Autodesk Fusion 360 part; units mm, degrees
(part 3 of 7)
sketch "Sketch8" plane through (0, 0, 0) normal (0, 0, 1) x (1, 0, 0)
  arc A0 (-0.8091, 5.4143) -> (-0.6399, 5.6347) centre (-0.8386, 5.6121) ccw
  arc A1 (0.6399, 5.6347) -> (0.8091, 5.4143) centre (0.8386, 5.6121) ccw
  line L0 (0.6399, 5.6347) -> (0.6786, 5.9756)
  spline S0 degree 5 poles (0.6786, 5.9756) (0.679, 5.9791) (0.6797, 5.9859) (0.6804, 5.9963) (0.6808, 6.0101) (0.6806, 6.0275) (0.6798, 6.0448) (0.6786, 6.0622) (0.6773, 6.0796) (0.6758, 6.0971) (0.6742, 6.1145) (0.6724, 6.132) (0.6704, 6.1495) (0.6682, 6.167) (0.6656, 6.1845) (0.6628, 6.202) (0.6598, 6.2196) (0.6566, 6.2371) (0.6532, 6.2546) (0.6497, 6.2722) (0.646, 6.2897) (0.6422, 6.3073) (0.6382, 6.3249) (0.634, 6.3424) (0.6297, 6.36) (0.6252, 6.3776) (0.6205, 6.3951) (0.6157, 6.4127) (0.6108, 6.4303) (0.6057, 6.4478) (0.6004, 6.4654) (0.595, 6.4829) (0.5895, 6.5005) (0.5838, 6.5181) (0.578, 6.5356) (0.5721, 6.5532) (0.566, 6.5707) (0.5598, 6.5882) (0.5535, 6.6058) (0.547, 6.6233) (0.5404, 6.6408) (0.5336, 6.6583) (0.5268, 6.6758) (0.5198, 6.6933) (0.5127, 6.7108) (0.5055, 6.7283) (0.4981, 6.7457) (0.4906, 6.7632) (0.483, 6.7806) (0.4753, 6.7981) (0.4675, 6.8155) (0.4595, 6.8329) (0.4514, 6.8503) (0.4432, 6.8677) (0.4349, 6.8851) (0.4265, 6.9024) (0.418, 6.9198) (0.4093, 6.9371) (0.4006, 6.9544) (0.3917, 6.9717) (0.3827, 6.989) (0.3736, 7.0063) (0.3644, 7.0235) (0.355, 7.0408) (0.3456, 7.058) (0.3361, 7.0752) (0.3264, 7.0924) (0.3167, 7.1095) (0.3068, 7.1267) (0.2968, 7.1438) (0.2867, 7.1609) (0.2786, 7.1746) (0.2724, 7.1848) (0.2683, 7.1917) (0.2662, 7.1951) knots 0 0 0 0 0 0 0.01428571 0.02857143 0.04285714 0.05714286 0.07142857 0.08571429 0.1 0.11428571 0.12857143 0.14285714 0.15714286 0.17142857 0.18571429 0.2 0.21428571 0.22857143 0.24285714 0.25714286 0.27142857 0.28571429 0.3 0.31428571 0.32857143 0.34285714 0.35714286 0.37142857 0.38571429 0.4 0.41428571 0.42857143 0.44285714 0.45714286 0.47142857 0.48571429 0.5 0.51428571 0.52857143 0.54285714 0.55714286 0.57142857 0.58571429 0.6 0.61428571 0.62857143 0.64285714 0.65714286 0.67142857 0.68571429 0.7 0.71428571 0.72857143 0.74285714 0.75714286 0.77142857 0.78571429 0.8 0.81428571 0.82857143 0.84285714 0.85714286 0.87142857 0.88571429 0.9 0.91428571 0.92857143 0.94285714 0.95714286 0.97142857 0.98571429 1 1 1 1 1 1
  line L1 (-0.6786, 5.9756) -> (-0.6399, 5.6347)
  spline S1 degree 5 poles (-0.6786, 5.9756) (-0.679, 5.9791) (-0.6797, 5.9859) (-0.6804, 5.9963) (-0.6808, 6.0101) (-0.6806, 6.0275) (-0.6798, 6.0448) (-0.6786, 6.0622) (-0.6773, 6.0796) (-0.6758, 6.0971) (-0.6742, 6.1145) (-0.6724, 6.132) (-0.6704, 6.1495) (-0.6682, 6.167) (-0.6656, 6.1845) (-0.6628, 6.202) (-0.6598, 6.2196) (-0.6566, 6.2371) (-0.6532, 6.2546) (-0.6497, 6.2722) (-0.646, 6.2897) (-0.6422, 6.3073) (-0.6382, 6.3249) (-0.634, 6.3424) (-0.6297, 6.36) (-0.6252, 6.3776) (-0.6205, 6.3951) (-0.6157, 6.4127) (-0.6108, 6.4303) (-0.6057, 6.4478) (-0.6004, 6.4654) (-0.595, 6.4829) (-0.5895, 6.5005) (-0.5838, 6.5181) (-0.578, 6.5356) (-0.5721, 6.5532) (-0.566, 6.5707) (-0.5598, 6.5882) (-0.5535, 6.6058) (-0.547, 6.6233) (-0.5404, 6.6408) (-0.5336, 6.6583) (-0.5268, 6.6758) (-0.5198, 6.6933) (-0.5127, 6.7108) (-0.5055, 6.7283) (-0.4981, 6.7457) (-0.4906, 6.7632) (-0.483, 6.7806) (-0.4753, 6.7981) (-0.4675, 6.8155) (-0.4595, 6.8329) (-0.4514, 6.8503) (-0.4432, 6.8677) (-0.4349, 6.8851) (-0.4265, 6.9024) (-0.418, 6.9198) (-0.4093, 6.9371) (-0.4006, 6.9544) (-0.3917, 6.9717) (-0.3827, 6.989) (-0.3736, 7.0063) (-0.3644, 7.0235) (-0.355, 7.0408) (-0.3456, 7.058) (-0.3361, 7.0752) (-0.3264, 7.0924) (-0.3167, 7.1095) (-0.3068, 7.1267) (-0.2968, 7.1438) (-0.2867, 7.1609) (-0.2786, 7.1746) (-0.2724, 7.1848) (-0.2683, 7.1917) (-0.2662, 7.1951) knots 0 0 0 0 0 0 0.01428571 0.02857143 0.04285714 0.05714286 0.07142857 0.08571429 0.1 0.11428571 0.12857143 0.14285714 0.15714286 0.17142857 0.18571429 0.2 0.21428571 0.22857143 0.24285714 0.25714286 0.27142857 0.28571429 0.3 0.31428571 0.32857143 0.34285714 0.35714286 0.37142857 0.38571429 0.4 0.41428571 0.42857143 0.44285714 0.45714286 0.47142857 0.48571429 0.5 0.51428571 0.52857143 0.54285714 0.55714286 0.57142857 0.58571429 0.6 0.61428571 0.62857143 0.64285714 0.65714286 0.67142857 0.68571429 0.7 0.71428571 0.72857143 0.74285714 0.75714286 0.77142857 0.78571429 0.8 0.81428571 0.82857143 0.84285714 0.85714286 0.87142857 0.88571429 0.9 0.91428571 0.92857143 0.94285714 0.95714286 0.97142857 0.98571429 1 1 1 1 1 1
  spline S2 degree 5 poles (-0.2662, 7.1951) (-0.2683, 7.1917) (-0.2724, 7.1848) (-0.2786, 7.1746) (-0.2867, 7.1609) (-0.2968, 7.1438) (-0.3068, 7.1267) (-0.3167, 7.1095) (-0.3264, 7.0924) (-0.3361, 7.0752) (-0.3456, 7.058) (-0.355, 7.0408) (-0.3644, 7.0235) (-0.3736, 7.0063) (-0.3827, 6.989) (-0.3917, 6.9717) (-0.4006, 6.9544) (-0.4093, 6.9371) (-0.418, 6.9198) (-0.4265, 6.9024) (-0.4349, 6.8851) (-0.4432, 6.8677) (-0.4514, 6.8503) (-0.4595, 6.8329) (-0.4675, 6.8155) (-0.4753, 6.7981) (-0.483, 6.7806) (-0.4906, 6.7632) (-0.4981, 6.7457) (-0.5055, 6.7283) (-0.5127, 6.7108) (-0.5198, 6.6933) (-0.5268, 6.6758) (-0.5336, 6.6583) (-0.5404, 6.6408) (-0.547, 6.6233) (-0.5535, 6.6058) (-0.5598, 6.5882) (-0.566, 6.5707) (-0.5721, 6.5532) (-0.578, 6.5356) (-0.5838, 6.5181) (-0.5895, 6.5005) (-0.595, 6.4829) (-0.6004, 6.4654) (-0.6057, 6.4478) (-0.6108, 6.4303) (-0.6157, 6.4127) (-0.6205, 6.3951) (-0.6252, 6.3776) (-0.6297, 6.36) (-0.634, 6.3424) (-0.6382, 6.3249) (-0.6422, 6.3073) (-0.646, 6.2897) (-0.6497, 6.2722) (-0.6532, 6.2546) (-0.6566, 6.2371) (-0.6598, 6.2196) (-0.6628, 6.202) (-0.6656, 6.1845) (-0.6682, 6.167) (-0.6704, 6.1495) (-0.6724, 6.132) (-0.6742, 6.1145) (-0.6758, 6.0971) (-0.6773, 6.0796) (-0.6786, 6.0622) (-0.6798, 6.0448) (-0.6806, 6.0275) (-0.6808, 6.0101) (-0.6804, 5.9963) (-0.6797, 5.9859) (-0.679, 5.9791) (-0.6786, 5.9756) knots -1 -1 -1 -1 -1 -1 -0.98571429 -0.97142857 -0.95714286 -0.94285714 -0.92857143 -0.91428571 -0.9 -0.88571429 -0.87142857 -0.85714286 -0.84285714 -0.82857143 -0.81428571 -0.8 -0.78571429 -0.77142857 -0.75714286 -0.74285714 -0.72857143 -0.71428571 -0.7 -0.68571429 -0.67142857 -0.65714286 -0.64285714 -0.62857143 -0.61428571 -0.6 -0.58571429 -0.57142857 -0.55714286 -0.54285714 -0.52857143 -0.51428571 -0.5 -0.48571429 -0.47142857 -0.45714286 -0.44285714 -0.42857143 -0.41428571 -0.4 -0.38571429 -0.37142857 -0.35714286 -0.34285714 -0.32857143 -0.31428571 -0.3 -0.28571429 -0.27142857 -0.25714286 -0.24285714 -0.22857143 -0.21428571 -0.2 -0.18571429 -0.17142857 -0.15714286 -0.14285714 -0.12857143 -0.11428571 -0.1 -0.08571429 -0.07142857 -0.05714286 -0.04285714 -0.02857143 -0.01428571 0 0 0 0 0 0
  spline S3 degree 5 poles (-0.2662, 7.1951) (-0.2683, 7.1917) (-0.2724, 7.1848) (-0.2786, 7.1746) (-0.2867, 7.1609) (-0.2968, 7.1438) (-0.3068, 7.1267) (-0.3167, 7.1095) (-0.3264, 7.0924) (-0.3361, 7.0752) (-0.3456, 7.058) (-0.355, 7.0408) (-0.3644, 7.0235) (-0.3736, 7.0063) (-0.3827, 6.989) (-0.3917, 6.9717) (-0.4006, 6.9544) (-0.4093, 6.9371) (-0.418, 6.9198) (-0.4265, 6.9024) (-0.4349, 6.8851) (-0.4432, 6.8677) (-0.4514, 6.8503) (-0.4595, 6.8329) (-0.4675, 6.8155) (-0.4753, 6.7981) (-0.483, 6.7806) (-0.4906, 6.7632) (-0.4981, 6.7457) (-0.5055, 6.7283) (-0.5127, 6.7108) (-0.5198, 6.6933) (-0.5268, 6.6758) (-0.5336, 6.6583) (-0.5404, 6.6408) (-0.547, 6.6233) (-0.5535, 6.6058) (-0.5598, 6.5882) (-0.566, 6.5707) (-0.5721, 6.5532) (-0.578, 6.5356) (-0.5838, 6.5181) (-0.5895, 6.5005) (-0.595, 6.4829) (-0.6004, 6.4654) (-0.6057, 6.4478) (-0.6108, 6.4303) (-0.6157, 6.4127) (-0.6205, 6.3951) (-0.6252, 6.3776) (-0.6297, 6.36) (-0.634, 6.3424) (-0.6382, 6.3249) (-0.6422, 6.3073) (-0.646, 6.2897) (-0.6497, 6.2722) (-0.6532, 6.2546) (-0.6566, 6.2371) (-0.6598, 6.2196) (-0.6628, 6.202) (-0.6656, 6.1845) (-0.6682, 6.167) (-0.6704, 6.1495) (-0.6724, 6.132) (-0.6742, 6.1145) (-0.6758, 6.0971) (-0.6773, 6.0796) (-0.6786, 6.0622) (-0.6798, 6.0448) (-0.6806, 6.0275) (-0.6808, 6.0101) (-0.6804, 5.9963) (-0.6797, 5.9859) (-0.679, 5.9791) (-0.6786, 5.9756) knots -1 -1 -1 -1 -1 -1 -0.98571429 -0.97142857 -0.95714286 -0.94285714 -0.92857143 -0.91428571 -0.9 -0.88571429 -0.87142857 -0.85714286 -0.84285714 -0.82857143 -0.81428571 -0.8 -0.78571429 -0.77142857 -0.75714286 -0.74285714 -0.72857143 -0.71428571 -0.7 -0.68571429 -0.67142857 -0.65714286 -0.64285714 -0.62857143 -0.61428571 -0.6 -0.58571429 -0.57142857 -0.55714286 -0.54285714 -0.52857143 -0.51428571 -0.5 -0.48571429 -0.47142857 -0.45714286 -0.44285714 -0.42857143 -0.41428571 -0.4 -0.38571429 -0.37142857 -0.35714286 -0.34285714 -0.32857143 -0.31428571 -0.3 -0.28571429 -0.27142857 -0.25714286 -0.24285714 -0.22857143 -0.21428571 -0.2 -0.18571429 -0.17142857 -0.15714286 -0.14285714 -0.12857143 -0.11428571 -0.1 -0.08571429 -0.07142857 -0.05714286 -0.04285714 -0.02857143 -0.01428571 0 0 0 0 0 0
  arc A2 (0.2662, 7.1951) -> (-0.2662, 7.1951) centre (0, 0) ccw
  arc A3 (-0.8091, 5.4143) -> (-0.6399, 5.6347) centre (-0.8386, 5.6121) ccw
  line L2 (-0.6399, 5.6347) -> (-0.6786, 5.9756)
  spline S4 degree 5 poles (-0.6786, 5.9756) (-0.679, 5.9791) (-0.6797, 5.9859) (-0.6804, 5.9963) (-0.6808, 6.0101) (-0.6806, 6.0275) (-0.6798, 6.0448) (-0.6786, 6.0622) (-0.6773, 6.0796) (-0.6758, 6.0971) (-0.6742, 6.1145) (-0.6724, 6.132) (-0.6704, 6.1495) (-0.6682, 6.167) (-0.6656, 6.1845) (-0.6628, 6.202) (-0.6598, 6.2196) (-0.6566, 6.2371) (-0.6532, 6.2546) (-0.6497, 6.2722) (-0.646, 6.2897) (-0.6422, 6.3073) (-0.6382, 6.3249) (-0.634, 6.3424) (-0.6297, 6.36) (-0.6252, 6.3776) (-0.6205, 6.3951) (-0.6157, 6.4127) (-0.6108, 6.4303) (-0.6057, 6.4478) (-0.6004, 6.4654) (-0.595, 6.4829) (-0.5895, 6.5005) (-0.5838, 6.5181) (-0.578, 6.5356) (-0.5721, 6.5532) (-0.566, 6.5707) (-0.5598, 6.5882) (-0.5535, 6.6058) (-0.547, 6.6233) (-0.5404, 6.6408) (-0.5336, 6.6583) (-0.5268, 6.6758) (-0.5198, 6.6933) (-0.5127, 6.7108) (-0.5055, 6.7283) (-0.4981, 6.7457) (-0.4906, 6.7632) (-0.483, 6.7806) (-0.4753, 6.7981) (-0.4675, 6.8155) (-0.4595, 6.8329) (-0.4514, 6.8503) (-0.4432, 6.8677) (-0.4349, 6.8851) (-0.4265, 6.9024) (-0.418, 6.9198) (-0.4093, 6.9371) (-0.4006, 6.9544) (-0.3917, 6.9717) (-0.3827, 6.989) (-0.3736, 7.0063) (-0.3644, 7.0235) (-0.355, 7.0408) (-0.3456, 7.058) (-0.3361, 7.0752) (-0.3264, 7.0924) (-0.3167, 7.1095) (-0.3068, 7.1267) (-0.2968, 7.1438) (-0.2867, 7.1609) (-0.2786, 7.1746) (-0.2724, 7.1848) (-0.2683, 7.1917) (-0.2662, 7.1951) knots 0 0 0 0 0 0 0.01428571 0.02857143 0.04285714 0.05714286 0.07142857 0.08571429 0.1 0.11428571 0.12857143 0.14285714 0.15714286 0.17142857 0.18571429 0.2 0.21428571 0.22857143 0.24285714 0.25714286 0.27142857 0.28571429 0.3 0.31428571 0.32857143 0.34285714 0.35714286 0.37142857 0.38571429 0.4 0.41428571 0.42857143 0.44285714 0.45714286 0.47142857 0.48571429 0.5 0.51428571 0.52857143 0.54285714 0.55714286 0.57142857 0.58571429 0.6 0.61428571 0.62857143 0.64285714 0.65714286 0.67142857 0.68571429 0.7 0.71428571 0.72857143 0.74285714 0.75714286 0.77142857 0.78571429 0.8 0.81428571 0.82857143 0.84285714 0.85714286 0.87142857 0.88571429 0.9 0.91428571 0.92857143 0.94285714 0.95714286 0.97142857 0.98571429 1 1 1 1 1 1
  arc A4 (0.2662, 7.1951) -> (-0.2662, 7.1951) centre (0, 0) ccw
  spline S5 degree 5 poles (0.6786, 5.9756) (0.679, 5.9791) (0.6797, 5.9859) (0.6804, 5.9963) (0.6808, 6.0101) (0.6806, 6.0275) (0.6798, 6.0448) (0.6786, 6.0622) (0.6773, 6.0796) (0.6758, 6.0971) (0.6742, 6.1145) (0.6724, 6.132) (0.6704, 6.1495) (0.6682, 6.167) (0.6656, 6.1845) (0.6628, 6.202) (0.6598, 6.2196) (0.6566, 6.2371) (0.6532, 6.2546) (0.6497, 6.2722) (0.646, 6.2897) (0.6422, 6.3073) (0.6382, 6.3249) (0.634, 6.3424) (0.6297, 6.36) (0.6252, 6.3776) (0.6205, 6.3951) (0.6157, 6.4127) (0.6108, 6.4303) (0.6057, 6.4478) (0.6004, 6.4654) (0.595, 6.4829) (0.5895, 6.5005) (0.5838, 6.5181) (0.578, 6.5356) (0.5721, 6.5532) (0.566, 6.5707) (0.5598, 6.5882) (0.5535, 6.6058) (0.547, 6.6233) (0.5404, 6.6408) (0.5336, 6.6583) (0.5268, 6.6758) (0.5198, 6.6933) (0.5127, 6.7108) (0.5055, 6.7283) (0.4981, 6.7457) (0.4906, 6.7632) (0.483, 6.7806) (0.4753, 6.7981) (0.4675, 6.8155) (0.4595, 6.8329) (0.4514, 6.8503) (0.4432, 6.8677) (0.4349, 6.8851) (0.4265, 6.9024) (0.418, 6.9198) (0.4093, 6.9371) (0.4006, 6.9544) (0.3917, 6.9717) (0.3827, 6.989) (0.3736, 7.0063) (0.3644, 7.0235) (0.355, 7.0408) (0.3456, 7.058) (0.3361, 7.0752) (0.3264, 7.0924) (0.3167, 7.1095) (0.3068, 7.1267) (0.2968, 7.1438) (0.2867, 7.1609) (0.2786, 7.1746) (0.2724, 7.1848) (0.2683, 7.1917) (0.2662, 7.1951) knots 0 0 0 0 0 0 0.01428571 0.02857143 0.04285714 0.05714286 0.07142857 0.08571429 0.1 0.11428571 0.12857143 0.14285714 0.15714286 0.17142857 0.18571429 0.2 0.21428571 0.22857143 0.24285714 0.25714286 0.27142857 0.28571429 0.3 0.31428571 0.32857143 0.34285714 0.35714286 0.37142857 0.38571429 0.4 0.41428571 0.42857143 0.44285714 0.45714286 0.47142857 0.48571429 0.5 0.51428571 0.52857143 0.54285714 0.55714286 0.57142857 0.58571429 0.6 0.61428571 0.62857143 0.64285714 0.65714286 0.67142857 0.68571429 0.7 0.71428571 0.72857143 0.74285714 0.75714286 0.77142857 0.78571429 0.8 0.81428571 0.82857143 0.84285714 0.85714286 0.87142857 0.88571429 0.9 0.91428571 0.92857143 0.94285714 0.95714286 0.97142857 0.98571429 1 1 1 1 1 1
  line L3 (0.6399, 5.6347) -> (0.6786, 5.9756)
  arc A5 (0.6399, 5.6347) -> (0.8091, 5.4143) centre (0.8386, 5.6121) ccw
  line L4 (-0.8091, 5.4143) -> (0.8091, 5.4143)
  constraint coincident A0.start A3.start
  constraint coincident A1.end A5.end
extrude "Extrude6" add sketch "Sketch8" along normal blind 4 separate body makes body 2
pattern_linear "R-Pattern1" count 18 spacing 2.5133 along (-1, 0, 0) both ways of bodies 2 makes body 3 at (17.3232, 5.4143, 2.6667) makes body 4 at (14.81, 5.4143, 1.3333) makes body 5 at (12.2967, 5.4143, 1.3333) makes body 6 at (9.7834, 5.4143, 1.3333) makes body 7 at (7.2701, 5.4143, 1.3333) makes body 8 at (4.7569, 5.4143, 1.3333) makes body 9 at (2.2436, 5.4143, 1.3333) makes body 10 at (-2.783, 5.4143, 1.3333) makes body 11 at (-5.2962, 5.4143, 1.3333) makes body 12 at (-7.8095, 5.4143, 1.3333) makes body 13 at (-10.3228, 5.4143, 1.3333) makes body 14 at (-12.8361, 5.4143, 1.3333) makes body 15 at (-15.3493, 5.4143, 1.3333) makes body 16 at (-17.8626, 5.4143, 2.6667) makes body 17 at (-20.3759, 5.4143, 2.6667) makes body 18 at (19.8365, 5.4143, 2.6667) makes body 19 at (-22.8892, 5.4143, 2.6667)
sketch "Sketch9" plane through (0, 0, 4) normal (0, 0, 1) x (-1, 0, 0)
  arc A0 (23.4285, -5.4143) -> (23.2594, -5.6347) centre (23.4581, -5.6121) ccw
  line L0 (23.4285, -5.4143) -> (21.8104, -5.4143)
  arc A1 (21.9796, -5.6347) -> (21.8104, -5.4143) centre (21.7809, -5.6121) ccw
  line L1 (21.9796, -5.6347) -> (21.9409, -5.9756)
  spline S0 degree 5 poles (21.9409, -5.9756) (21.9405, -5.9791) (21.9398, -5.9859) (21.939, -5.9963) (21.9386, -6.0101) (21.9389, -6.0275) (21.9397, -6.0448) (21.9408, -6.0622) (21.9422, -6.0796) (21.9436, -6.0971) (21.9453, -6.1145) (21.947, -6.132) (21.949, -6.1495) (21.9513, -6.167) (21.9538, -6.1845) (21.9566, -6.202) (21.9597, -6.2196) (21.9629, -6.2371) (21.9662, -6.2546) (21.9698, -6.2722) (21.9734, -6.2897) (21.9773, -6.3073) (21.9813, -6.3249) (21.9854, -6.3424) (21.9898, -6.36) (21.9943, -6.3776) (21.9989, -6.3951) (22.0037, -6.4127) (22.0087, -6.4303) (22.0138, -6.4478) (22.019, -6.4654) (22.0244, -6.4829) (22.03, -6.5005) (22.0356, -6.5181) (22.0414, -6.5356) (22.0474, -6.5532) (22.0535, -6.5707) (22.0597, -6.5882) (22.066, -6.6058) (22.0725, -6.6233) (22.0791, -6.6408) (22.0858, -6.6583) (22.0927, -6.6758) (22.0997, -6.6933) (22.1068, -6.7108) (22.114, -6.7283) (22.1214, -6.7457) (22.1288, -6.7632) (22.1364, -6.7806) (22.1442, -6.7981) (22.152, -6.8155) (22.16, -6.8329) (22.168, -6.8503) (22.1762, -6.8677) (22.1845, -6.8851) (22.193, -6.9024) (22.2015, -6.9198) (22.2101, -6.9371) (22.2189, -6.9544) (22.2278, -6.9717) (22.2368, -6.989) (22.2459, -7.0063) (22.2551, -7.0235) (22.2644, -7.0408) (22.2739, -7.058) (22.2834, -7.0752) (22.2931, -7.0924) (22.3028, -7.1095) (22.3127, -7.1267) (22.3227, -7.1438) (22.3327, -7.1609) (22.3409, -7.1746) (22.347, -7.1848) (22.3512, -7.1917) (22.3532, -7.1951) knots 0 0 0 0 0 0 0.01428571 0.02857143 0.04285714 0.05714286 0.07142857 0.08571429 0.1 0.11428571 0.12857143 0.14285714 0.15714286 0.17142857 0.18571429 0.2 0.21428571 0.22857143 0.24285714 0.25714286 0.27142857 0.28571429 0.3 0.31428571 0.32857143 0.34285714 0.35714286 0.37142857 0.38571429 0.4 0.41428571 0.42857143 0.44285714 0.45714286 0.47142857 0.48571429 0.5 0.51428571 0.52857143 0.54285714 0.55714286 0.57142857 0.58571429 0.6 0.61428571 0.62857143 0.64285714 0.65714286 0.67142857 0.68571429 0.7 0.71428571 0.72857143 0.74285714 0.75714286 0.77142857 0.78571429 0.8 0.81428571 0.82857143 0.84285714 0.85714286 0.87142857 0.88571429 0.9 0.91428571 0.92857143 0.94285714 0.95714286 0.97142857 0.98571429 1 1 1 1 1 1
  arc A2 (22.3532, -7.1951) -> (22.8857, -7.1951) centre (22.6195, 0) ccw
  spline S1 degree 5 poles (22.8857, -7.1951) (22.8878, -7.1917) (22.8919, -7.1848) (22.898, -7.1746) (22.9062, -7.1609) (22.9163, -7.1438) (22.9263, -7.1267) (22.9361, -7.1095) (22.9459, -7.0924) (22.9555, -7.0752) (22.9651, -7.058) (22.9745, -7.0408) (22.9838, -7.0235) (22.993, -7.0063) (23.0022, -6.989) (23.0111, -6.9717) (23.02, -6.9544) (23.0288, -6.9371) (23.0374, -6.9198) (23.046, -6.9024) (23.0544, -6.8851) (23.0627, -6.8677) (23.0709, -6.8503) (23.079, -6.8329) (23.0869, -6.8155) (23.0948, -6.7981) (23.1025, -6.7806) (23.1101, -6.7632) (23.1176, -6.7457) (23.1249, -6.7283) (23.1322, -6.7108) (23.1393, -6.6933) (23.1463, -6.6758) (23.1531, -6.6583) (23.1598, -6.6408) (23.1664, -6.6233) (23.1729, -6.6058) (23.1793, -6.5882) (23.1855, -6.5707) (23.1916, -6.5532) (23.1975, -6.5356) (23.2033, -6.5181) (23.209, -6.5005) (23.2145, -6.4829) (23.2199, -6.4654) (23.2251, -6.4478) (23.2302, -6.4303) (23.2352, -6.4127) (23.24, -6.3951) (23.2447, -6.3776) (23.2492, -6.36) (23.2535, -6.3424) (23.2577, -6.3249) (23.2617, -6.3073) (23.2655, -6.2897) (23.2692, -6.2722) (23.2727, -6.2546) (23.2761, -6.2371) (23.2793, -6.2196) (23.2823, -6.202) (23.2851, -6.1845) (23.2876, -6.167) (23.2899, -6.1495) (23.2919, -6.132) (23.2937, -6.1145) (23.2953, -6.0971) (23.2968, -6.0796) (23.2981, -6.0622) (23.2993, -6.0448) (23.3001, -6.0275) (23.3003, -6.0101) (23.2999, -5.9963) (23.2992, -5.9859) (23.2985, -5.9791) (23.2981, -5.9756) knots -1 -1 -1 -1 -1 -1 -0.98571429 -0.97142857 -0.95714286 -0.94285714 -0.92857143 -0.91428571 -0.9 -0.88571429 -0.87142857 -0.85714286 -0.84285714 -0.82857143 -0.81428571 -0.8 -0.78571429 -0.77142857 -0.75714286 -0.74285714 -0.72857143 -0.71428571 -0.7 -0.68571429 -0.67142857 -0.65714286 -0.64285714 -0.62857143 -0.61428571 -0.6 -0.58571429 -0.57142857 -0.55714286 -0.54285714 -0.52857143 -0.51428571 -0.5 -0.48571429 -0.47142857 -0.45714286 -0.44285714 -0.42857143 -0.41428571 -0.4 -0.38571429 -0.37142857 -0.35714286 -0.34285714 -0.32857143 -0.31428571 -0.3 -0.28571429 -0.27142857 -0.25714286 -0.24285714 -0.22857143 -0.21428571 -0.2 -0.18571429 -0.17142857 -0.15714286 -0.14285714 -0.12857143 -0.11428571 -0.1 -0.08571429 -0.07142857 -0.05714286 -0.04285714 -0.02857143 -0.01428571 0 0 0 0 0 0
  line L2 (23.2981, -5.9756) -> (23.2594, -5.6347)
  line L3 (23.4285, -5.4143) -> (-20.9152, -5.4143)
  line L4 (-20.9152, -5.4143) -> (-20.9152, -3.6143)
  line L5 (-20.9152, -3.6143) -> (23.4285, -3.6143)
  line L6 (23.4285, -3.6143) -> (23.4285, -5.4143)
  point P0 (23.4285, -5.4143)
  point P1 (-20.9152, -5.4143)
  dimension "d25" = 1.8
  constraint perpendicular L3 L4
  constraint parallel L3 L5
  constraint parallel L4 L6
  constraint coincident P1 L3.end
  constraint parallel L0 L3
  constraint coincident P0 A0.start
  measures "d25" distance of P0 L5.end
extrude "Extrude7" add sketch "Sketch9" against normal up to surface (4 mm away) contours L0 L3 L4 L5 L6 bodies 2 18 3 4 5 6 7 8 9 10 11 12 13 14 15 16 17 19
copy_body "CopyPasteBodies1" bodies 2 makes body 20
move_body "Move1" bodies 20 to x (1, 0, 0) y (0, 1, 0) z (0, 0, 1) at (3.7199, -2.3078, -0.6071)
extrude "Extrude8" add 1 faces at (24.6351, 2.5065, 2.0595) along direction (1, 0, 0) blind 5 on bodies 20 bodies 20
sketch "Sketch10" plane through (0, 1.3065, 0) normal (0, -1, 0) x (1, 0, 0)
  line L0 (-19.7086, -0.6071) -> (29.6351, -0.6071)
  line L1 (29.6351, -0.6071) -> (29.6351, 3.3929)
  line L2 (29.6351, 3.3929) -> (-19.7086, 3.3929)
  line L3 (-19.7086, 3.3929) -> (-19.7086, -0.6071)
  line L4 (29.6351, -0.6071) -> (24.6351, -0.6071)
  line L5 (24.6351, -0.6071) -> (24.6351, 3.3929)
  line L6 (24.6351, 3.3929) -> (29.6351, 3.3929)
  line L7 (29.6351, 3.3929) -> (29.6351, -0.6071)
  dimension "d30" = 5
  constraint horizontal L4
  constraint vertical L5
  constraint horizontal L6
  constraint vertical L7
  constraint coincident L0.end L1.start
  measures "d30" distance of L0.end L4.end
extrude "Extrude9" add sketch "Sketch10" against normal blind 25 contours L0 L1 L2 L4 L5 L6 L7 bodies 20
sketch "Sketch11" plane through (0, 0, 3.3929) normal (0, 0, 1) x (-1, 0, 0)
  arc A0 (-23.017, -3.1065) -> (-23.1862, -3.3269) centre (-22.9875, -3.3043) ccw
  line L0 (-23.017, -3.1065) -> (-22.1219, -3.1065)
  arc A1 (-21.9527, -3.3269) -> (-22.1219, -3.1065) centre (-22.1514, -3.3043) ccw
  line L1 (-21.9527, -3.3269) -> (-21.9914, -3.6679)
  spline S0 degree 5 poles (-21.9914, -3.6679) (-21.9918, -3.6713) (-21.9925, -3.6782) (-21.9932, -3.6885) (-21.9936, -3.7024) (-21.9934, -3.7197) (-21.9926, -3.7371) (-21.9914, -3.7545) (-21.9901, -3.7719) (-21.9886, -3.7893) (-21.987, -3.8068) (-21.9852, -3.8243) (-21.9832, -3.8417) (-21.981, -3.8592) (-21.9784, -3.8768) (-21.9756, -3.8943) (-21.9726, -3.9118) (-21.9694, -3.9293) (-21.966, -3.9469) (-21.9625, -3.9644) (-21.9588, -3.982) (-21.955, -3.9995) (-21.951, -4.0171) (-21.9469, -4.0347) (-21.9425, -4.0522) (-21.938, -4.0698) (-21.9333, -4.0874) (-21.9285, -4.1049) (-21.9236, -4.1225) (-21.9185, -4.1401) (-21.9132, -4.1576) (-21.9078, -4.1752) (-21.9023, -4.1928) (-21.8966, -4.2103) (-21.8908, -4.2279) (-21.8849, -4.2454) (-21.8788, -4.2629) (-21.8726, -4.2805) (-21.8663, -4.298) (-21.8598, -4.3155) (-21.8532, -4.3331) (-21.8465, -4.3506) (-21.8396, -4.3681) (-21.8326, -4.3856) (-21.8255, -4.403) (-21.8183, -4.4205) (-21.8109, -4.438) (-21.8034, -4.4554) (-21.7958, -4.4729) (-21.7881, -4.4903) (-21.7803, -4.5077) (-21.7723, -4.5252) (-21.7642, -4.5426) (-21.7561, -4.5599) (-21.7477, -4.5773) (-21.7393, -4.5947) (-21.7308, -4.612) (-21.7221, -4.6293) (-21.7134, -4.6467) (-21.7045, -4.664) (-21.6955, -4.6813) (-21.6864, -4.6985) (-21.6772, -4.7158) (-21.6678, -4.733) (-21.6584, -4.7502) (-21.6489, -4.7674) (-21.6392, -4.7846) (-21.6295, -4.8018) (-21.6196, -4.8189) (-21.6096, -4.8361) (-21.5995, -4.8532) (-21.5914, -4.8668) (-21.5852, -4.8771) (-21.5811, -4.8839) (-21.579, -4.8873) knots 0 0 0 0 0 0 0.01428571 0.02857143 0.04285714 0.05714286 0.07142857 0.08571429 0.1 0.11428571 0.12857143 0.14285714 0.15714286 0.17142857 0.18571429 0.2 0.21428571 0.22857143 0.24285714 0.25714286 0.27142857 0.28571429 0.3 0.31428571 0.32857143 0.34285714 0.35714286 0.37142857 0.38571429 0.4 0.41428571 0.42857143 0.44285714 0.45714286 0.47142857 0.48571429 0.5 0.51428571 0.52857143 0.54285714 0.55714286 0.57142857 0.58571429 0.6 0.61428571 0.62857143 0.64285714 0.65714286 0.67142857 0.68571429 0.7 0.71428571 0.72857143 0.74285714 0.75714286 0.77142857 0.78571429 0.8 0.81428571 0.82857143 0.84285714 0.85714286 0.87142857 0.88571429 0.9 0.91428571 0.92857143 0.94285714 0.95714286 0.97142857 0.98571429 1 1 1 1 1 1
  arc A2 (-21.579, -4.8873) -> (-21.0466, -4.8873) centre (-21.3128, 2.3078) ccw
  spline S1 degree 5 poles (-21.0466, -4.8873) (-21.0445, -4.8839) (-21.0404, -4.8771) (-21.0342, -4.8668) (-21.0261, -4.8532) (-21.016, -4.8361) (-21.006, -4.8189) (-20.9962, -4.8018) (-20.9864, -4.7846) (-20.9767, -4.7674) (-20.9672, -4.7502) (-20.9578, -4.733) (-20.9484, -4.7158) (-20.9392, -4.6985) (-20.9301, -4.6813) (-20.9211, -4.664) (-20.9123, -4.6467) (-20.9035, -4.6293) (-20.8948, -4.612) (-20.8863, -4.5947) (-20.8779, -4.5773) (-20.8696, -4.5599) (-20.8614, -4.5426) (-20.8533, -4.5252) (-20.8453, -4.5077) (-20.8375, -4.4903) (-20.8298, -4.4729) (-20.8222, -4.4554) (-20.8147, -4.438) (-20.8073, -4.4205) (-20.8001, -4.403) (-20.793, -4.3856) (-20.786, -4.3681) (-20.7792, -4.3506) (-20.7724, -4.3331) (-20.7658, -4.3155) (-20.7594, -4.298) (-20.753, -4.2805) (-20.7468, -4.2629) (-20.7407, -4.2454) (-20.7348, -4.2279) (-20.729, -4.2103) (-20.7233, -4.1928) (-20.7178, -4.1752) (-20.7124, -4.1576) (-20.7071, -4.1401) (-20.702, -4.1225) (-20.6971, -4.1049) (-20.6923, -4.0874) (-20.6876, -4.0698) (-20.6831, -4.0522) (-20.6788, -4.0347) (-20.6746, -4.0171) (-20.6706, -3.9995) (-20.6668, -3.982) (-20.6631, -3.9644) (-20.6596, -3.9469) (-20.6562, -3.9293) (-20.653, -3.9118) (-20.65, -3.8943) (-20.6472, -3.8768) (-20.6446, -3.8592) (-20.6424, -3.8417) (-20.6404, -3.8243) (-20.6386, -3.8068) (-20.637, -3.7893) (-20.6355, -3.7719) (-20.6342, -3.7545) (-20.633, -3.7371) (-20.6322, -3.7197) (-20.632, -3.7024) (-20.6324, -3.6885) (-20.6331, -3.6782) (-20.6338, -3.6713) (-20.6342, -3.6679) knots -1 -1 -1 -1 -1 -1 -0.98571429 -0.97142857 -0.95714286 -0.94285714 -0.92857143 -0.91428571 -0.9 -0.88571429 -0.87142857 -0.85714286 -0.84285714 -0.82857143 -0.81428571 -0.8 -0.78571429 -0.77142857 -0.75714286 -0.74285714 -0.72857143 -0.71428571 -0.7 -0.68571429 -0.67142857 -0.65714286 -0.64285714 -0.62857143 -0.61428571 -0.6 -0.58571429 -0.57142857 -0.55714286 -0.54285714 -0.52857143 -0.51428571 -0.5 -0.48571429 -0.47142857 -0.45714286 -0.44285714 -0.42857143 -0.41428571 -0.4 -0.38571429 -0.37142857 -0.35714286 -0.34285714 -0.32857143 -0.31428571 -0.3 -0.28571429 -0.27142857 -0.25714286 -0.24285714 -0.22857143 -0.21428571 -0.2 -0.18571429 -0.17142857 -0.15714286 -0.14285714 -0.12857143 -0.11428571 -0.1 -0.08571429 -0.07142857 -0.05714286 -0.04285714 -0.02857143 -0.01428571 0 0 0 0 0 0
  line L2 (-20.6342, -3.6679) -> (-20.6729, -3.3269)
  arc A3 (-20.5037, -3.1065) -> (-20.6729, -3.3269) centre (-20.4742, -3.3043) ccw
  line L3 (-20.5037, -3.1065) -> (-19.6086, -3.1065)
  arc A4 (-19.4394, -3.3269) -> (-19.6086, -3.1065) centre (-19.6381, -3.3043) ccw
  line L4 (-19.4394, -3.3269) -> (-19.4781, -3.6679)
  spline S2 degree 5 poles (-19.4781, -3.6679) (-19.4785, -3.6713) (-19.4792, -3.6782) (-19.48, -3.6885) (-19.4804, -3.7024) (-19.4801, -3.7197) (-19.4793, -3.7371) (-19.4782, -3.7545) (-19.4768, -3.7719) (-19.4753, -3.7893) (-19.4737, -3.8068) (-19.472, -3.8243) (-19.47, -3.8417) (-19.4677, -3.8592) (-19.4652, -3.8768) (-19.4624, -3.8943) (-19.4593, -3.9118) (-19.4561, -3.9293) (-19.4528, -3.9469) (-19.4492, -3.9644) (-19.4456, -3.982) (-19.4417, -3.9995) (-19.4377, -4.0171) (-19.4336, -4.0347) (-19.4292, -4.0522) (-19.4247, -4.0698) (-19.4201, -4.0874) (-19.4153, -4.1049) (-19.4103, -4.1225) (-19.4052, -4.1401) (-19.4, -4.1576) (-19.3946, -4.1752) (-19.389, -4.1928) (-19.3834, -4.2103) (-19.3776, -4.2279) (-19.3716, -4.2454) (-19.3655, -4.2629) (-19.3593, -4.2805) (-19.353, -4.298) (-19.3465, -4.3155) (-19.3399, -4.3331) (-19.3332, -4.3506) (-19.3263, -4.3681) (-19.3193, -4.3856) (-19.3122, -4.403) (-19.305, -4.4205) (-19.2976, -4.438) (-19.2902, -4.4554) (-19.2826, -4.4729) (-19.2748, -4.4903) (-19.267, -4.5077) (-19.259, -4.5252) (-19.251, -4.5426) (-19.2428, -4.5599) (-19.2345, -4.5773) (-19.226, -4.5947) (-19.2175, -4.612) (-19.2089, -4.6293) (-19.2001, -4.6467) (-19.1912, -4.664) (-19.1822, -4.6813) (-19.1731, -4.6985) (-19.1639, -4.7158) (-19.1546, -4.733) (-19.1451, -4.7502) (-19.1356, -4.7674) (-19.1259, -4.7846) (-19.1162, -4.8018) (-19.1063, -4.8189) (-19.0963, -4.8361) (-19.0863, -4.8532) (-19.0781, -4.8668) (-19.072, -4.8771) (-19.0678, -4.8839) (-19.0658, -4.8873) knots 0 0 0 0 0 0 0.01428571 0.02857143 0.04285714 0.05714286 0.07142857 0.08571429 0.1 0.11428571 0.12857143 0.14285714 0.15714286 0.17142857 0.18571429 0.2 0.21428571 0.22857143 0.24285714 0.25714286 0.27142857 0.28571429 0.3 0.31428571 0.32857143 0.34285714 0.35714286 0.37142857 0.38571429 0.4 0.41428571 0.42857143 0.44285714 0.45714286 0.47142857 0.48571429 0.5 0.51428571 0.52857143 0.54285714 0.55714286 0.57142857 0.58571429 0.6 0.61428571 0.62857143 0.64285714 0.65714286 0.67142857 0.68571429 0.7 0.71428571 0.72857143 0.74285714 0.75714286 0.77142857 0.78571429 0.8 0.81428571 0.82857143 0.84285714 0.85714286 0.87142857 0.88571429 0.9 0.91428571 0.92857143 0.94285714 0.95714286 0.97142857 0.98571429 1 1 1 1 1 1
  arc A5 (-19.0658, -4.8873) -> (-18.5333, -4.8873) centre (-18.7995, 2.3078) ccw
  spline S3 degree 5 poles (-18.5333, -4.8873) (-18.5312, -4.8839) (-18.5271, -4.8771) (-18.521, -4.8668) (-18.5128, -4.8532) (-18.5027, -4.8361) (-18.4927, -4.8189) (-18.4829, -4.8018) (-18.4731, -4.7846) (-18.4635, -4.7674) (-18.4539, -4.7502) (-18.4445, -4.733) (-18.4352, -4.7158) (-18.426, -4.6985) (-18.4168, -4.6813) (-18.4079, -4.664) (-18.399, -4.6467) (-18.3902, -4.6293) (-18.3816, -4.612) (-18.373, -4.5947) (-18.3646, -4.5773) (-18.3563, -4.5599) (-18.3481, -4.5426) (-18.34, -4.5252) (-18.3321, -4.5077) (-18.3242, -4.4903) (-18.3165, -4.4729) (-18.3089, -4.4554) (-18.3014, -4.438) (-18.2941, -4.4205) (-18.2868, -4.403) (-18.2797, -4.3856) (-18.2727, -4.3681) (-18.2659, -4.3506) (-18.2592, -4.3331) (-18.2526, -4.3155) (-18.2461, -4.298) (-18.2397, -4.2805) (-18.2335, -4.2629) (-18.2274, -4.2454) (-18.2215, -4.2279) (-18.2157, -4.2103) (-18.21, -4.1928) (-18.2045, -4.1752) (-18.1991, -4.1576) (-18.1939, -4.1401) (-18.1888, -4.1225) (-18.1838, -4.1049) (-18.179, -4.0874) (-18.1743, -4.0698) (-18.1698, -4.0522) (-18.1655, -4.0347) (-18.1613, -4.0171) (-18.1573, -3.9995) (-18.1535, -3.982) (-18.1498, -3.9644) (-18.1463, -3.9469) (-18.1429, -3.9293) (-18.1397, -3.9118) (-18.1367, -3.8943) (-18.1339, -3.8768) (-18.1314, -3.8592) (-18.1291, -3.8417) (-18.1271, -3.8243) (-18.1253, -3.8068) (-18.1237, -3.7893) (-18.1222, -3.7719) (-18.1209, -3.7545) (-18.1197, -3.7371) (-18.1189, -3.7197) (-18.1187, -3.7024) (-18.1191, -3.6885) (-18.1198, -3.6782) (-18.1205, -3.6713) (-18.1209, -3.6679) knots -1 -1 -1 -1 -1 -1 -0.98571429 -0.97142857 -0.95714286 -0.94285714 -0.92857143 -0.91428571 -0.9 -0.88571429 -0.87142857 -0.85714286 -0.84285714 -0.82857143 -0.81428571 -0.8 -0.78571429 -0.77142857 -0.75714286 -0.74285714 -0.72857143 -0.71428571 -0.7 -0.68571429 -0.67142857 -0.65714286 -0.64285714 -0.62857143 -0.61428571 -0.6 -0.58571429 -0.57142857 -0.55714286 -0.54285714 -0.52857143 -0.51428571 -0.5 -0.48571429 -0.47142857 -0.45714286 -0.44285714 -0.42857143 -0.41428571 -0.4 -0.38571429 -0.37142857 -0.35714286 -0.34285714 -0.32857143 -0.31428571 -0.3 -0.28571429 -0.27142857 -0.25714286 -0.24285714 -0.22857143 -0.21428571 -0.2 -0.18571429 -0.17142857 -0.15714286 -0.14285714 -0.12857143 -0.11428571 -0.1 -0.08571429 -0.07142857 -0.05714286 -0.04285714 -0.02857143 -0.01428571 0 0 0 0 0 0
  line L5 (-18.1209, -3.6679) -> (-18.1596, -3.3269)
  arc A6 (-17.9905, -3.1065) -> (-18.1596, -3.3269) centre (-17.9609, -3.3043) ccw
  line L6 (-17.9905, -3.1065) -> (-17.0953, -3.1065)
  arc A7 (-16.9262, -3.3269) -> (-17.0953, -3.1065) centre (-17.1249, -3.3043) ccw
  line L7 (-16.9262, -3.3269) -> (-16.9649, -3.6679)
  spline S4 degree 5 poles (-16.9649, -3.6679) (-16.9653, -3.6713) (-16.9659, -3.6782) (-16.9667, -3.6885) (-16.9671, -3.7024) (-16.9668, -3.7197) (-16.966, -3.7371) (-16.9649, -3.7545) (-16.9635, -3.7719) (-16.9621, -3.7893) (-16.9605, -3.8068) (-16.9587, -3.8243) (-16.9567, -3.8417) (-16.9544, -3.8592) (-16.9519, -3.8768) (-16.9491, -3.8943) (-16.9461, -3.9118) (-16.9429, -3.9293) (-16.9395, -3.9469) (-16.936, -3.9644) (-16.9323, -3.982) (-16.9285, -3.9995) (-16.9245, -4.0171) (-16.9203, -4.0347) (-16.916, -4.0522) (-16.9115, -4.0698) (-16.9068, -4.0874) (-16.902, -4.1049) (-16.897, -4.1225) (-16.8919, -4.1401) (-16.8867, -4.1576) (-16.8813, -4.1752) (-16.8758, -4.1928) (-16.8701, -4.2103) (-16.8643, -4.2279) (-16.8583, -4.2454) (-16.8523, -4.2629) (-16.8461, -4.2805) (-16.8397, -4.298) (-16.8332, -4.3155) (-16.8266, -4.3331) (-16.8199, -4.3506) (-16.813, -4.3681) (-16.8061, -4.3856) (-16.799, -4.403) (-16.7917, -4.4205) (-16.7844, -4.438) (-16.7769, -4.4554) (-16.7693, -4.4729) (-16.7616, -4.4903) (-16.7537, -4.5077) (-16.7458, -4.5252) (-16.7377, -4.5426) (-16.7295, -4.5599) (-16.7212, -4.5773) (-16.7128, -4.5947) (-16.7042, -4.612) (-16.6956, -4.6293) (-16.6868, -4.6467) (-16.6779, -4.664) (-16.6689, -4.6813) (-16.6598, -4.6985) (-16.6506, -4.7158) (-16.6413, -4.733) (-16.6319, -4.7502) (-16.6223, -4.7674) (-16.6127, -4.7846) (-16.6029, -4.8018) (-16.593, -4.8189) (-16.5831, -4.8361) (-16.573, -4.8532) (-16.5648, -4.8668) (-16.5587, -4.8771) (-16.5545, -4.8839) (-16.5525, -4.8873) knots 0 0 0 0 0 0 0.01428571 0.02857143 0.04285714 0.05714286 0.07142857 0.08571429 0.1 0.11428571 0.12857143 0.14285714 0.15714286 0.17142857 0.18571429 0.2 0.21428571 0.22857143 0.24285714 0.25714286 0.27142857 0.28571429 0.3 0.31428571 0.32857143 0.34285714 0.35714286 0.37142857 0.38571429 0.4 0.41428571 0.42857143 0.44285714 0.45714286 0.47142857 0.48571429 0.5 0.51428571 0.52857143 0.54285714 0.55714286 0.57142857 0.58571429 0.6 0.61428571 0.62857143 0.64285714 0.65714286 0.67142857 0.68571429 0.7 0.71428571 0.72857143 0.74285714 0.75714286 0.77142857 0.78571429 0.8 0.81428571 0.82857143 0.84285714 0.85714286 0.87142857 0.88571429 0.9 0.91428571 0.92857143 0.94285714 0.95714286 0.97142857 0.98571429 1 1 1 1 1 1
  arc A8 (-16.5525, -4.8873) -> (-16.02, -4.8873) centre (-16.2863, 2.3078) ccw
  spline S5 degree 5 poles (-16.02, -4.8873) (-16.018, -4.8839) (-16.0138, -4.8771) (-16.0077, -4.8668) (-15.9995, -4.8532) (-15.9894, -4.8361) (-15.9795, -4.8189) (-15.9696, -4.8018) (-15.9598, -4.7846) (-15.9502, -4.7674) (-15.9407, -4.7502) (-15.9312, -4.733) (-15.9219, -4.7158) (-15.9127, -4.6985) (-15.9036, -4.6813) (-15.8946, -4.664) (-15.8857, -4.6467) (-15.8769, -4.6293) (-15.8683, -4.612) (-15.8597, -4.5947) (-15.8513, -4.5773) (-15.843, -4.5599) (-15.8348, -4.5426) (-15.8267, -4.5252) (-15.8188, -4.5077) (-15.811, -4.4903) (-15.8032, -4.4729) (-15.7956, -4.4554) (-15.7882, -4.438) (-15.7808, -4.4205) (-15.7736, -4.403) (-15.7665, -4.3856) (-15.7595, -4.3681) (-15.7526, -4.3506) (-15.7459, -4.3331) (-15.7393, -4.3155) (-15.7328, -4.298) (-15.7265, -4.2805) (-15.7202, -4.2629) (-15.7142, -4.2454) (-15.7082, -4.2279) (-15.7024, -4.2103) (-15.6967, -4.1928) (-15.6912, -4.1752) (-15.6858, -4.1576) (-15.6806, -4.1401) (-15.6755, -4.1225) (-15.6705, -4.1049) (-15.6657, -4.0874) (-15.6611, -4.0698) (-15.6565, -4.0522) (-15.6522, -4.0347) (-15.648, -4.0171) (-15.644, -3.9995) (-15.6402, -3.982) (-15.6365, -3.9644) (-15.633, -3.9469) (-15.6297, -3.9293) (-15.6265, -3.9118) (-15.6234, -3.8943) (-15.6206, -3.8768) (-15.6181, -3.8592) (-15.6158, -3.8417) (-15.6138, -3.8243) (-15.612, -3.8068) (-15.6104, -3.7893) (-15.609, -3.7719) (-15.6076, -3.7545) (-15.6065, -3.7371) (-15.6057, -3.7197) (-15.6054, -3.7024) (-15.6058, -3.6885) (-15.6066, -3.6782) (-15.6073, -3.6713) (-15.6076, -3.6679) knots -1 -1 -1 -1 -1 -1 -0.98571429 -0.97142857 -0.95714286 -0.94285714 -0.92857143 -0.91428571 -0.9 -0.88571429 -0.87142857 -0.85714286 -0.84285714 -0.82857143 -0.81428571 -0.8 -0.78571429 -0.77142857 -0.75714286 -0.74285714 -0.72857143 -0.71428571 -0.7 -0.68571429 -0.67142857 -0.65714286 -0.64285714 -0.62857143 -0.61428571 -0.6 -0.58571429 -0.57142857 -0.55714286 -0.54285714 -0.52857143 -0.51428571 -0.5 -0.48571429 -0.47142857 -0.45714286 -0.44285714 -0.42857143 -0.41428571 -0.4 -0.38571429 -0.37142857 -0.35714286 -0.34285714 -0.32857143 -0.31428571 -0.3 -0.28571429 -0.27142857 -0.25714286 -0.24285714 -0.22857143 -0.21428571 -0.2 -0.18571429 -0.17142857 -0.15714286 -0.14285714 -0.12857143 -0.11428571 -0.1 -0.08571429 -0.07142857 -0.05714286 -0.04285714 -0.02857143 -0.01428571 0 0 0 0 0 0
  line L8 (-15.6076, -3.6679) -> (-15.6464, -3.3269)
  arc A9 (-15.4772, -3.1065) -> (-15.6464, -3.3269) centre (-15.4476, -3.3043) ccw
  line L9 (-15.4772, -3.1065) -> (-14.582, -3.1065)
  arc A10 (-14.4129, -3.3269) -> (-14.582, -3.1065) centre (-14.6116, -3.3043) ccw
  line L10 (-14.4129, -3.3269) -> (-14.4516, -3.6679)
  spline S6 degree 5 poles (-14.4516, -3.6679) (-14.452, -3.6713) (-14.4527, -3.6782) (-14.4534, -3.6885) (-14.4538, -3.7024) (-14.4536, -3.7197) (-14.4528, -3.7371) (-14.4516, -3.7545) (-14.4503, -3.7719) (-14.4488, -3.7893) (-14.4472, -3.8068) (-14.4454, -3.8243) (-14.4434, -3.8417) (-14.4411, -3.8592) (-14.4386, -3.8768) (-14.4358, -3.8943) (-14.4328, -3.9118) (-14.4296, -3.9293) (-14.4262, -3.9469) (-14.4227, -3.9644) (-14.419, -3.982) (-14.4152, -3.9995) (-14.4112, -4.0171) (-14.407, -4.0347) (-14.4027, -4.0522) (-14.3982, -4.0698) (-14.3935, -4.0874) (-14.3887, -4.1049) (-14.3837, -4.1225) (-14.3786, -4.1401) (-14.3734, -4.1576) (-14.368, -4.1752) (-14.3625, -4.1928) (-14.3568, -4.2103) (-14.351, -4.2279) (-14.3451, -4.2454) (-14.339, -4.2629) (-14.3328, -4.2805) (-14.3264, -4.298) (-14.32, -4.3155) (-14.3134, -4.3331) (-14.3066, -4.3506) (-14.2998, -4.3681) (-14.2928, -4.3856) (-14.2857, -4.403) (-14.2784, -4.4205) (-14.2711, -4.438) (-14.2636, -4.4554) (-14.256, -4.4729) (-14.2483, -4.4903) (-14.2405, -4.5077) (-14.2325, -4.5252) (-14.2244, -4.5426) (-14.2162, -4.5599) (-14.2079, -4.5773) (-14.1995, -4.5947) (-14.191, -4.612) (-14.1823, -4.6293) (-14.1735, -4.6467) (-14.1647, -4.664) (-14.1557, -4.6813) (-14.1466, -4.6985) (-14.1374, -4.7158) (-14.128, -4.733) (-14.1186, -4.7502) (-14.109, -4.7674) (-14.0994, -4.7846) (-14.0896, -4.8018) (-14.0798, -4.8189) (-14.0698, -4.8361) (-14.0597, -4.8532) (-14.0516, -4.8668) (-14.0454, -4.8771) (-14.0413, -4.8839) (-14.0392, -4.8873) knots 0 0 0 0 0 0 0.01428571 0.02857143 0.04285714 0.05714286 0.07142857 0.08571429 0.1 0.11428571 0.12857143 0.14285714 0.15714286 0.17142857 0.18571429 0.2 0.21428571 0.22857143 0.24285714 0.25714286 0.27142857 0.28571429 0.3 0.31428571 0.32857143 0.34285714 0.35714286 0.37142857 0.38571429 0.4 0.41428571 0.42857143 0.44285714 0.45714286 0.47142857 0.48571429 0.5 0.51428571 0.52857143 0.54285714 0.55714286 0.57142857 0.58571429 0.6 0.61428571 0.62857143 0.64285714 0.65714286 0.67142857 0.68571429 0.7 0.71428571 0.72857143 0.74285714 0.75714286 0.77142857 0.78571429 0.8 0.81428571 0.82857143 0.84285714 0.85714286 0.87142857 0.88571429 0.9 0.91428571 0.92857143 0.94285714 0.95714286 0.97142857 0.98571429 1 1 1 1 1 1
  arc A11 (-14.0392, -4.8873) -> (-13.5068, -4.8873) centre (-13.773, 2.3078) ccw
  spline S7 degree 5 poles (-13.5068, -4.8873) (-13.5047, -4.8839) (-13.5006, -4.8771) (-13.4944, -4.8668) (-13.4863, -4.8532) (-13.4762, -4.8361) (-13.4662, -4.8189) (-13.4563, -4.8018) (-13.4466, -4.7846) (-13.4369, -4.7674) (-13.4274, -4.7502) (-13.4179, -4.733) (-13.4086, -4.7158) (-13.3994, -4.6985) (-13.3903, -4.6813) (-13.3813, -4.664) (-13.3724, -4.6467) (-13.3637, -4.6293) (-13.355, -4.612) (-13.3465, -4.5947) (-13.338, -4.5773) (-13.3297, -4.5599) (-13.3215, -4.5426) (-13.3135, -4.5252) (-13.3055, -4.5077) (-13.2977, -4.4903) (-13.29, -4.4729) (-13.2824, -4.4554) (-13.2749, -4.438) (-13.2675, -4.4205) (-13.2603, -4.403) (-13.2532, -4.3856) (-13.2462, -4.3681) (-13.2393, -4.3506) (-13.2326, -4.3331) (-13.226, -4.3155) (-13.2195, -4.298) (-13.2132, -4.2805) (-13.207, -4.2629) (-13.2009, -4.2454) (-13.1949, -4.2279) (-13.1891, -4.2103) (-13.1835, -4.1928) (-13.1779, -4.1752) (-13.1726, -4.1576) (-13.1673, -4.1401) (-13.1622, -4.1225) (-13.1573, -4.1049) (-13.1524, -4.0874) (-13.1478, -4.0698) (-13.1433, -4.0522) (-13.1389, -4.0347) (-13.1348, -4.0171) (-13.1308, -3.9995) (-13.1269, -3.982) (-13.1233, -3.9644) (-13.1198, -3.9469) (-13.1164, -3.9293) (-13.1132, -3.9118) (-13.1102, -3.8943) (-13.1074, -3.8768) (-13.1048, -3.8592) (-13.1025, -3.8417) (-13.1005, -3.8243) (-13.0988, -3.8068) (-13.0972, -3.7893) (-13.0957, -3.7719) (-13.0944, -3.7545) (-13.0932, -3.7371) (-13.0924, -3.7197) (-13.0921, -3.7024) (-13.0926, -3.6885) (-13.0933, -3.6782) (-13.094, -3.6713) (-13.0944, -3.6679) knots -1 -1 -1 -1 -1 -1 -0.98571429 -0.97142857 -0.95714286 -0.94285714 -0.92857143 -0.91428571 -0.9 -0.88571429 -0.87142857 -0.85714286 -0.84285714 -0.82857143 -0.81428571 -0.8 -0.78571429 -0.77142857 -0.75714286 -0.74285714 -0.72857143 -0.71428571 -0.7 -0.68571429 -0.67142857 -0.65714286 -0.64285714 -0.62857143 -0.61428571 -0.6 -0.58571429 -0.57142857 -0.55714286 -0.54285714 -0.52857143 -0.51428571 -0.5 -0.48571429 -0.47142857 -0.45714286 -0.44285714 -0.42857143 -0.41428571 -0.4 -0.38571429 -0.37142857 -0.35714286 -0.34285714 -0.32857143 -0.31428571 -0.3 -0.28571429 -0.27142857 -0.25714286 -0.24285714 -0.22857143 -0.21428571 -0.2 -0.18571429 -0.17142857 -0.15714286 -0.14285714 -0.12857143 -0.11428571 -0.1 -0.08571429 -0.07142857 -0.05714286 -0.04285714 -0.02857143 -0.01428571 0 0 0 0 0 0
  line L11 (-13.0944, -3.6679) -> (-13.1331, -3.3269)
  arc A12 (-12.9639, -3.1065) -> (-13.1331, -3.3269) centre (-12.9344, -3.3043) ccw
  line L12 (-12.9639, -3.1065) -> (-12.0688, -3.1065)
  arc A13 (-11.8996, -3.3269) -> (-12.0688, -3.1065) centre (-12.0983, -3.3043) ccw
  line L13 (-11.8996, -3.3269) -> (-11.9383, -3.6679)
  spline S8 degree 5 poles (-11.9383, -3.6679) (-11.9387, -3.6713) (-11.9394, -3.6782) (-11.9401, -3.6885) (-11.9405, -3.7024) (-11.9403, -3.7197) (-11.9395, -3.7371) (-11.9383, -3.7545) (-11.937, -3.7719) (-11.9355, -3.7893) (-11.9339, -3.8068) (-11.9321, -3.8243) (-11.9301, -3.8417) (-11.9279, -3.8592) (-11.9253, -3.8768) (-11.9225, -3.8943) (-11.9195, -3.9118) (-11.9163, -3.9293) (-11.9129, -3.9469) (-11.9094, -3.9644) (-11.9058, -3.982) (-11.9019, -3.9995) (-11.8979, -4.0171) (-11.8938, -4.0347) (-11.8894, -4.0522) (-11.8849, -4.0698) (-11.8802, -4.0874) (-11.8754, -4.1049) (-11.8705, -4.1225) (-11.8654, -4.1401) (-11.8601, -4.1576) (-11.8547, -4.1752) (-11.8492, -4.1928) (-11.8436, -4.2103) (-11.8377, -4.2279) (-11.8318, -4.2454) (-11.8257, -4.2629) (-11.8195, -4.2805) (-11.8132, -4.298) (-11.8067, -4.3155) (-11.8001, -4.3331) (-11.7934, -4.3506) (-11.7865, -4.3681) (-11.7795, -4.3856) (-11.7724, -4.403) (-11.7652, -4.4205) (-11.7578, -4.438) (-11.7503, -4.4554) (-11.7427, -4.4729) (-11.735, -4.4903) (-11.7272, -4.5077) (-11.7192, -4.5252) (-11.7111, -4.5426) (-11.703, -4.5599) (-11.6946, -4.5773) (-11.6862, -4.5947) (-11.6777, -4.612) (-11.669, -4.6293) (-11.6603, -4.6467) (-11.6514, -4.664) (-11.6424, -4.6813) (-11.6333, -4.6985) (-11.6241, -4.7158) (-11.6148, -4.733) (-11.6053, -4.7502) (-11.5958, -4.7674) (-11.5861, -4.7846) (-11.5764, -4.8018) (-11.5665, -4.8189) (-11.5565, -4.8361) (-11.5464, -4.8532) (-11.5383, -4.8668) (-11.5321, -4.8771) (-11.528, -4.8839) (-11.5259, -4.8873) knots 0 0 0 0 0 0 0.01428571 0.02857143 0.04285714 0.05714286 0.07142857 0.08571429 0.1 0.11428571 0.12857143 0.14285714 0.15714286 0.17142857 0.18571429 0.2 0.21428571 0.22857143 0.24285714 0.25714286 0.27142857 0.28571429 0.3 0.31428571 0.32857143 0.34285714 0.35714286 0.37142857 0.38571429 0.4 0.41428571 0.42857143 0.44285714 0.45714286 0.47142857 0.48571429 0.5 0.51428571 0.52857143 0.54285714 0.55714286 0.57142857 0.58571429 0.6 0.61428571 0.62857143 0.64285714 0.65714286 0.67142857 0.68571429 0.7 0.71428571 0.72857143 0.74285714 0.75714286 0.77142857 0.78571429 0.8 0.81428571 0.82857143 0.84285714 0.85714286 0.87142857 0.88571429 0.9 0.91428571 0.92857143 0.94285714 0.95714286 0.97142857 0.98571429 1 1 1 1 1 1
  arc A14 (-11.5259, -4.8873) -> (-10.9935, -4.8873) centre (-11.2597, 2.3078) ccw
  spline S9 degree 5 poles (-10.9935, -4.8873) (-10.9914, -4.8839) (-10.9873, -4.8771) (-10.9811, -4.8668) (-10.973, -4.8532) (-10.9629, -4.8361) (-10.9529, -4.8189) (-10.9431, -4.8018) (-10.9333, -4.7846) (-10.9236, -4.7674) (-10.9141, -4.7502) (-10.9047, -4.733) (-10.8953, -4.7158) (-10.8861, -4.6985) (-10.877, -4.6813) (-10.868, -4.664) (-10.8592, -4.6467) (-10.8504, -4.6293) (-10.8417, -4.612) (-10.8332, -4.5947) (-10.8248, -4.5773) (-10.8165, -4.5599) (-10.8083, -4.5426) (-10.8002, -4.5252) (-10.7922, -4.5077) (-10.7844, -4.4903) (-10.7767, -4.4729) (-10.7691, -4.4554) (-10.7616, -4.438) (-10.7542, -4.4205) (-10.747, -4.403) (-10.7399, -4.3856) (-10.7329, -4.3681) (-10.7261, -4.3506) (-10.7193, -4.3331) (-10.7127, -4.3155) (-10.7063, -4.298) (-10.6999, -4.2805) (-10.6937, -4.2629) (-10.6876, -4.2454) (-10.6817, -4.2279) (-10.6759, -4.2103) (-10.6702, -4.1928) (-10.6647, -4.1752) (-10.6593, -4.1576) (-10.654, -4.1401) (-10.6489, -4.1225) (-10.644, -4.1049) (-10.6392, -4.0874) (-10.6345, -4.0698) (-10.63, -4.0522) (-10.6257, -4.0347) (-10.6215, -4.0171) (-10.6175, -3.9995) (-10.6137, -3.982) (-10.61, -3.9644) (-10.6065, -3.9469) (-10.6031, -3.9293) (-10.5999, -3.9118) (-10.5969, -3.8943) (-10.5941, -3.8768) (-10.5915, -3.8592) (-10.5893, -3.8417) (-10.5873, -3.8243) (-10.5855, -3.8068) (-10.5839, -3.7893) (-10.5824, -3.7719) (-10.5811, -3.7545) (-10.5799, -3.7371) (-10.5791, -3.7197) (-10.5789, -3.7024) (-10.5793, -3.6885) (-10.58, -3.6782) (-10.5807, -3.6713) (-10.5811, -3.6679) knots -1 -1 -1 -1 -1 -1 -0.98571429 -0.97142857 -0.95714286 -0.94285714 -0.92857143 -0.91428571 -0.9 -0.88571429 -0.87142857 -0.85714286 -0.84285714 -0.82857143 -0.81428571 -0.8 -0.78571429 -0.77142857 -0.75714286 -0.74285714 -0.72857143 -0.71428571 -0.7 -0.68571429 -0.67142857 -0.65714286 -0.64285714 -0.62857143 -0.61428571 -0.6 -0.58571429 -0.57142857 -0.55714286 -0.54285714 -0.52857143 -0.51428571 -0.5 -0.48571429 -0.47142857 -0.45714286 -0.44285714 -0.42857143 -0.41428571 -0.4 -0.38571429 -0.37142857 -0.35714286 -0.34285714 -0.32857143 -0.31428571 -0.3 -0.28571429 -0.27142857 -0.25714286 -0.24285714 -0.22857143 -0.21428571 -0.2 -0.18571429 -0.17142857 -0.15714286 -0.14285714 -0.12857143 -0.11428571 -0.1 -0.08571429 -0.07142857 -0.05714286 -0.04285714 -0.02857143 -0.01428571 0 0 0 0 0 0
  line L14 (-10.5811, -3.6679) -> (-10.6198, -3.3269)
  arc A15 (-10.4507, -3.1065) -> (-10.6198, -3.3269) centre (-10.4211, -3.3043) ccw
  line L15 (-10.4507, -3.1065) -> (-9.5555, -3.1065)
  arc A16 (-9.3863, -3.3269) -> (-9.5555, -3.1065) centre (-9.5851, -3.3043) ccw
  line L16 (-9.3863, -3.3269) -> (-9.425, -3.6679)
  spline S10 degree 5 poles (-9.425, -3.6679) (-9.4254, -3.6713) (-9.4261, -3.6782) (-9.4269, -3.6885) (-9.4273, -3.7024) (-9.427, -3.7197) (-9.4262, -3.7371) (-9.4251, -3.7545) (-9.4237, -3.7719) (-9.4223, -3.7893) (-9.4207, -3.8068) (-9.4189, -3.8243) (-9.4169, -3.8417) (-9.4146, -3.8592) (-9.4121, -3.8768) (-9.4093, -3.8943) (-9.4062, -3.9118) (-9.403, -3.9293) (-9.3997, -3.9469) (-9.3961, -3.9644) (-9.3925, -3.982) (-9.3886, -3.9995) (-9.3847, -4.0171) (-9.3805, -4.0347) (-9.3761, -4.0522) (-9.3716, -4.0698) (-9.367, -4.0874) (-9.3622, -4.1049) (-9.3572, -4.1225) (-9.3521, -4.1401) (-9.3469, -4.1576) (-9.3415, -4.1752) (-9.3359, -4.1928) (-9.3303, -4.2103) (-9.3245, -4.2279) (-9.3185, -4.2454) (-9.3124, -4.2629) (-9.3062, -4.2805) (-9.2999, -4.298) (-9.2934, -4.3155) (-9.2868, -4.3331) (-9.2801, -4.3506) (-9.2732, -4.3681) (-9.2662, -4.3856) (-9.2591, -4.403) (-9.2519, -4.4205) (-9.2445, -4.438) (-9.2371, -4.4554) (-9.2295, -4.4729) (-9.2217, -4.4903) (-9.2139, -4.5077) (-9.2059, -4.5252) (-9.1979, -4.5426) (-9.1897, -4.5599) (-9.1814, -4.5773) (-9.1729, -4.5947) (-9.1644, -4.612) (-9.1558, -4.6293) (-9.147, -4.6467) (-9.1381, -4.664) (-9.1291, -4.6813) (-9.12, -4.6985) (-9.1108, -4.7158) (-9.1015, -4.733) (-9.092, -4.7502) (-9.0825, -4.7674) (-9.0728, -4.7846) (-9.0631, -4.8018) (-9.0532, -4.8189) (-9.0432, -4.8361) (-9.0332, -4.8532) (-9.025, -4.8668) (-9.0189, -4.8771) (-9.0147, -4.8839) (-9.0127, -4.8873) knots 0 0 0 0 0 0 0.01428571 0.02857143 0.04285714 0.05714286 0.07142857 0.08571429 0.1 0.11428571 0.12857143 0.14285714 0.15714286 0.17142857 0.18571429 0.2 0.21428571 0.22857143 0.24285714 0.25714286 0.27142857 0.28571429 0.3 0.31428571 0.32857143 0.34285714 0.35714286 0.37142857 0.38571429 0.4 0.41428571 0.42857143 0.44285714 0.45714286 0.47142857 0.48571429 0.5 0.51428571 0.52857143 0.54285714 0.55714286 0.57142857 0.58571429 0.6 0.61428571 0.62857143 0.64285714 0.65714286 0.67142857 0.68571429 0.7 0.71428571 0.72857143 0.74285714 0.75714286 0.77142857 0.78571429 0.8 0.81428571 0.82857143 0.84285714 0.85714286 0.87142857 0.88571429 0.9 0.91428571 0.92857143 0.94285714 0.95714286 0.97142857 0.98571429 1 1 1 1 1 1
  arc A17 (-9.0127, -4.8873) -> (-8.4802, -4.8873) centre (-8.7464, 2.3078) ccw